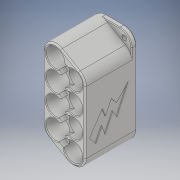
# Autodesk Inventor part: AUX_battery_pack
Saved by Autodesk Inventor 2019 (Build 230136000, 136)
## iProperties
Created: 2019-11-13
Part Number: AUX_battery_pack
Material: Generic
Document SubType Name: Modeling
Designer: steve
Density: 1 g/cm^3
Appearance: Default
Author: steve
Autodesk Inventor part; units mm, degrees
ref_plane "YZ Plane" through (0, 0, 0) normal (1, 0, 0) x (0, 1, 0)
ref_plane "XZ Plane" through (0, 0, 0) normal (0, 1, 0) x (-1, 0, 0)
ref_plane "XY Plane" through (0, 0, 0) normal (0, 0, 1) x (1, 0, 0)
sketch "Sketch1" plane through (0, 0, 0) normal (0, 0, 1) x (1, 0, 0)
  circle A0 centre (0, 60) radius 13.45
  circle A1 centre (0, 30) radius 13.45
  circle A2 centre (0, 0) radius 13.45
  circle A3 centre (0, -30) radius 13.45
  line L0 (0, 60) -> (0, -30) construction
  circle A4 centre (25.980762, 45) radius 13.45
  circle A5 centre (25.980762, 15) radius 13.45
  circle A6 centre (25.980762, -15) radius 13.45
  circle A7 centre (25.980762, -45) radius 13.45
  line L1 (25.980762, 45) -> (25.980762, -45) construction
  line L2 (-17.45, 60) -> (-17.45, -30)
  line L3 (43.430762, 45) -> (43.430762, -45)
  arc A8 (17.255762, -60.112143) -> (43.430762, -45) centre (25.980762, -45) ccw
  line L4 (8.725, 75.112143) -> (34.705762, 60.112143)
  line L5 (17.255762, -60.112143) -> (-8.725, -45.112143)
  arc A9 (43.430762, 45) -> (34.705762, 60.112143) centre (25.980762, 45) ccw
  arc A10 (8.725, 75.112143) -> (-17.45, 60) centre (0, 60) ccw
  arc A11 (-17.45, -30) -> (-8.725, -45.112143) centre (0, -30) ccw
  dimension "d0" = 30
  dimension "d1" = 30
  dimension "d2" = 30
  dimension "d3" = 30
  dimension "d4" = 30
  dimension "d5" = 30
  dimension "d6" = 26.9
  dimension "d7" = 30
  dimension "d8" = 30
  dimension "d10" = 17.45
  dimension "d11" = 17.45
  constraints: 13 end point, 12 centre point, 8 point on circle, 7 equal radius, 7 tangent, 4 point on line, 4 vertical, 1 coincident, 1 parallel
  measures "d0" distance of A1.centre L0.start
  measures "d1" distance of A2.centre A1.centre
  measures "d2" distance of L0.end A2.centre
  measures "d3" distance of A5.centre L1.start
  measures "d4" distance of A6.centre A5.centre
  measures "d5" distance of L1.end A6.centre
  measures "d6" diameter of A0
  measures "d7" distance of L1.start L0.start
  measures "d8" distance of A1.centre L1.start
  measures "d10" distance from line of L2 L0.start
  measures "d11" distance from line of L3 L1.start
extrude "Extrusion1" add sketch "Sketch1" along normal blind 70
sketch "Sketch2" plane through (0, 0, 0) normal (0, 0, -1) x (-1, 0, 0)
  line L0 (8.725, -45.112143) -> (-17.255762, -60.112143)
  arc A0 (8.725, -45.112143) -> (17.45, -30) centre (0, -30) ccw
  line L1 (17.45, 60) -> (17.45, -30)
  arc A1 (-43.430762, -45) -> (-17.255762, -60.112143) centre (-25.980762, -45) ccw
  line L2 (-43.430762, -45) -> (-43.430762, 45)
  arc A2 (-34.705762, 60.112143) -> (-43.430762, 45) centre (-25.980762, 45) ccw
  line L3 (-34.705762, 60.112143) -> (-8.725, 75.112143)
  arc A3 (17.45, 60) -> (-8.725, 75.112143) centre (0, 60) ccw
  point P0 (0, 0)
extrude "Extrusion2" add sketch "Sketch2" along normal blind 5
sketch "Sketch3" plane through (0, 0, -5) normal (0, 0, -1) x (-1, 0, 0)
  circle A0 centre (0, -30) radius 13.45
  circle A1 centre (-25.980762, -45) radius 13.45
  circle A2 centre (-25.980762, -15) radius 13.45
  circle A3 centre (0, 0) radius 13.45
  circle A4 centre (-25.980762, 15) radius 13.45
  circle A5 centre (-25.980762, 45) radius 13.45
  circle A6 centre (0, 30) radius 13.45
  circle A7 centre (0, 60) radius 13.45
  line L0 (0, -30) -> (-25.980762, -45) construction
  line L1 (-3.75, -23.504809) -> (-29.730762, -38.504809)
  line L2 (-22.230762, -51.495191) -> (3.75, -36.495191)
  arc A8 (3.75, -36.495191) -> (-3.75, -23.504809) centre (0, -30) ccw
  arc A9 (-29.730762, -38.504809) -> (-22.230762, -51.495191) centre (-25.980762, -45) ccw
  line L3 (-25.980762, -15) -> (0, 0) construction
  line L4 (-29.730762, -8.504809) -> (-3.75, 6.495191)
  line L5 (3.75, -6.495191) -> (-22.230762, -21.495191)
  arc A10 (-29.730762, -8.504809) -> (-22.230762, -21.495191) centre (-25.980762, -15) ccw
  arc A11 (3.75, -6.495191) -> (-3.75, 6.495191) centre (0, 0) ccw
  line L6 (-25.980762, 15) -> (0, 30) construction
  line L7 (-22.230762, 8.504809) -> (3.75, 23.504809)
  line L8 (-3.75, 36.495191) -> (-29.730762, 21.495191)
  arc A12 (-29.730762, 21.495191) -> (-22.230762, 8.504809) centre (-25.980762, 15) ccw
  arc A13 (3.75, 23.504809) -> (-3.75, 36.495191) centre (0, 30) ccw
  line L9 (-25.980762, 45) -> (0, 60) construction
  line L10 (-29.730762, 51.495191) -> (-3.75, 66.495191)
  line L11 (3.75, 53.504809) -> (-22.230762, 38.504809)
  arc A14 (-29.730762, 51.495191) -> (-22.230762, 38.504809) centre (-25.980762, 45) ccw
  arc A15 (3.75, 53.504809) -> (-3.75, 66.495191) centre (0, 60) ccw
  point P0 (-12.990381, -37.5)
  point P1 (-12.990381, -7.5)
  point P2 (-12.990381, 22.5)
  point P3 (-12.990381, 52.5)
  dimension "d16" = 15
  constraints: 32 end point, 16 point on circle, 16 tangent, 8 centre point, 7 parallel, 4 midpoint, 3 equal radius, 1 coincident
  measures "d16" distance between parallel lines of L1 L2
extrude "Extrusion3" cut sketch "Sketch3" against normal blind 8 contours L1 A8 L2 A0 | A0 L2 A1 L1 | A1 L2 A9 L1 | A2 L5 A10 L4 | A2 L4 A3 L5 | L4 A11 L5 A3 | A4 L7 A12 L8 | A4 L8 A6 L7 | L8 A13 L7 A6 | A5 L11 A14 L10 | A5 L10 A7 L11 | L10 A15 L11 A7 picked at (-4.12012, -31.767735) picked at (-21.936079, -43.065881) picked at (-21.936079, -13.065881) picked at (-4.12012, -1.767735) picked at (-21.936079, 16.934119) picked at (-4.12012, 28.232265) picked at (-21.936079, 46.934119) picked at (-4.12012, 58.232265)
sketch "Sketch5" plane through (0, 0, 70) normal (0, 0, 1) x (1, 0, 0)
  circle A0 centre (25.980762, 45) radius 13.45
  circle A1 centre (0, 30) radius 13.45
  circle A2 centre (25.980762, 15) radius 13.45
  circle A3 centre (25.980762, -15) radius 13.45
  circle A4 centre (0, -30) radius 13.45
  line L0 (25.980762, 45) -> (0, 30) construction
  line L1 (22.230762, 51.495191) -> (-3.75, 36.495191)
  line L2 (3.75, 23.504809) -> (29.730762, 38.504809)
  arc A5 (29.730762, 38.504809) -> (22.230762, 51.495191) centre (25.980762, 45) ccw
  arc A6 (-3.75, 36.495191) -> (3.75, 23.504809) centre (0, 30) ccw
  arc A7 (3.75, 66.495191) -> (-3.75, 53.504809) centre (0, 60) ccw
  line L3 (25.980762, 15) -> (0, 0) construction
  line L4 (22.230762, 21.495191) -> (-3.75, 6.495191)
  line L5 (3.75, -6.495191) -> (29.730762, 8.504809)
  arc A8 (29.730762, 8.504809) -> (22.230762, 21.495191) centre (25.980762, 15) ccw
  arc A9 (-3.75, 6.495191) -> (3.75, -6.495191) centre (0, 0) ccw
  line L6 (25.980762, -15) -> (0, -30) construction
  line L7 (22.230762, -8.504809) -> (-3.75, -23.504809)
  line L8 (3.75, -36.495191) -> (29.730762, -21.495191)
  arc A10 (29.730762, -21.495191) -> (22.230762, -8.504809) centre (25.980762, -15) ccw
  arc A11 (-3.75, -23.504809) -> (3.75, -36.495191) centre (0, -30) ccw
  point P0 (12.990381, 37.5)
  point P1 (12.990381, 7.5)
  point P2 (12.990381, -22.5)
  constraints: 24 end point, 12 point on circle, 12 tangent, 6 centre point, 4 parallel, 3 equal radius, 3 midpoint
extrude "Extrusion5" cut sketch "Sketch5" against normal blind 8 contours L1 A5 L2 A0 | A0 L2 A1 L1 | A1 L2 A6 L1 | L4 A8 L5 A2 | A2 L5 A9 L4 | L7 A10 L8 A3 | A3 L8 A4 L7 | A4 L8 A11 L7 picked at (21.860642, 43.232265) picked at (4.044683, 31.934119) picked at (21.860642, 13.232265) picked at (21.860642, -16.767735) picked at (4.044683, -28.065881)
sketch "Sketch6" plane through (0, 0, -5) normal (0, 0, -1) x (-1, 0, 0)
  arc A0 (17.45, 60) -> (-8.725, 75.112143) centre (0, 60) ccw
  line L0 (0, 77.45) -> (-25.980762, 77.45)
  line L1 (-43.430762, -45) -> (-43.430762, 45)
  line L2 (-43.430762, 60) -> (-43.430762, 45)
  arc A1 (-43.430762, -45) -> (-17.255762, -60.112143) centre (-25.980762, -45) ccw
  line L3 (-25.980762, -62.45) -> (0, -62.45)
  arc A2 (8.725, -45.112143) -> (17.45, -30) centre (0, -30) ccw
  line L4 (17.45, -45) -> (17.45, -30)
  arc A3 (0, -62.45) -> (17.45, -45) centre (0, -45) ccw
  arc A4 (-25.980762, 77.45) -> (-43.430762, 60) centre (-25.980762, 60) ccw
  arc A5 (17.45, 60) -> (-8.725, 75.112143) centre (0, 60) ccw
  circle A6 centre (-32.980762, 68) radius 3.5
  circle A7 centre (7, -53) radius 3.5
  arc A8 (-34.705762, 60.112143) -> (-43.430762, 45) centre (-25.980762, 45) ccw
  line L5 (-8.725, 75.112143) -> (-34.705762, 60.112143)
  line L6 (-17.255762, -60.112143) -> (8.725, -45.112143)
  point P0 (0, 0)
  dimension "d25" = 7
  dimension "d26" = 8
  dimension "d27" = 8
  dimension "d28" = 7
  dimension "d29" = 7
  constraints: 8 end point, 7 tangent, 6 point on circle, 4 centre point, 3 equal radius, 2 horizontal, 1 collinear, 1 perpendicular
  measures "d25" horizontal distance of A4.centre A6.centre
  measures "d26" vertical distance of A4.centre A6.centre
  measures "d27" vertical distance of A3.centre A7.centre
  measures "d28" horizontal distance of A3.centre A7.centre
  measures "d29" diameter of A6
extrude "Extrusion6" add sketch "Sketch6" against normal blind 8
chamfer "Chamfer1" distance 1 angle 45 6 edges at (12.9904, 77.45, 3) (38.3198, 72.339, 3) (43.4308, 52.5, 3) (-12.339, -57.339, 3) (12.9904, -62.45, 3) (-17.45, -37.5, 3)
chamfer "Chamfer2" distance 2 angle 45 16 edges at (-17.45, 15, 70) (-15.1121, -38.725, 70) (4.2654, -52.6121, 70) (34.7058, -60.1121, 70) (43.4308, 0, 70) (41.0929, 53.725, 70) (21.7154, 67.6121, 70) (-8.725, 75.1121, 70) (-17.45, 7.5, -5) (-12.339, 72.339, -5) (12.9904, 77.45, -5) (38.3198, 72.339, -5) (43.4308, 7.5, -5) (38.3198, -57.339, -5) (12.9904, -62.45, -5) (-12.339, -57.339, -5)
fillet "Fillet1" radius 1 11 edges at (12.5308, -45, 70) (-11.648, -36.725, 70) (-11.648, -6.725, 70) (33.0974, -26.413, 70) (26.4374, -1.5578, 70) (33.0974, 3.587, 70) (26.4374, 28.4422, 70) (-11.648, 23.275, 70) (-13.45, 60, 70) (33.0974, 33.587, 70) (26.4374, 58.4422, 70)
sketch "Sketch7" plane through (43.430762, 45, 2) normal (1, 0, 0) x (0, 0, -1)
  line L0 (-52.607783, -78.238394) -> (-61.826281, -67.020119)
  line L1 (-61.826281, -67.020119) -> (-43.228078, -39.325419)
  line L2 (-43.228078, -39.325419) -> (-38.644697, -50.847251)
  line L3 (-30.271785, -32.948873) -> (-22.700002, -42.051274)
  line L4 (-22.700002, -42.051274) -> (-5.868775, -23.837274)
  line L5 (-28.217884, -49.779066) -> (-22.387126, -60.267263)
  line L6 (-22.387126, -60.267263) -> (-5.868775, -23.837274)
  line L7 (-28.217884, -49.779066) -> (-39.286312, -73.570399)
  line L8 (-39.286312, -73.570399) -> (-43.874505, -60.51306)
  line L9 (-43.874505, -60.51306) -> (-52.607783, -78.238394)
  line L10 (-38.644697, -50.847251) -> (-30.271785, -32.948873)
  point P0 (2, -45)
  point P1 (23.5, -4.5)
  dimension "d39" = 33.36
  dimension "d40" = 14.52
  dimension "d41" = 19.76
  dimension "d42" = 13.84
  dimension "d43" = 26.24
  dimension "d44" = 19.76
  dimension "d45" = 12.4
  dimension "d46" = 11.84
  dimension "d47" = 24.8
  dimension "d48" = 40
  dimension "d49" = 12
  constraints: 22 end point
  measures "d39" distance of L0.end L1.end
  measures "d40" distance of L0.start L0.end
  measures "d41" distance of L8.end L0.start
  measures "d42" distance of L7.end L8.end
  measures "d43" distance of L5.start L7.end
  measures "d44" distance of L2.end L3.start
  measures "d45" distance of L1.end L2.end
  measures "d46" distance of L3.start L3.end
  measures "d47" distance of L3.end L4.end
  measures "d48" distance of L5.end L4.end
  measures "d49" distance of L5.start L5.end
extrude "Extrusion7" cut sketch "Sketch7" against normal blind 1
sketch "Sketch8" plane through (0, 0, 70) normal (0, 0, 1) x (1, 0, 0)
  arc A0 (5.91899, -17.922415) -> (13.41899, -30.912796) centre (0, -30) ccw
  arc A1 (20.061772, -27.077585) -> (12.561772, -14.087204) centre (25.980762, -15) ccw
  arc A2 (5.91899, 12.077585) -> (13.41899, -0.912796) centre (0, 0) ccw
  arc A3 (20.061772, 2.922415) -> (12.561772, 15.912796) centre (25.980762, 15) ccw
  arc A4 (5.91899, 42.077585) -> (13.41899, 29.087204) centre (0, 30) ccw
  arc A5 (20.061772, 32.922415) -> (12.561772, 45.912796) centre (25.980762, 45) ccw
  circle A6 centre (0, 60) radius 13.45
  circle A7 centre (25.980762, -45) radius 13.45
  arc A8 (22.230762, 38.504809) -> (29.730762, 51.495191) centre (25.980762, 45) ccw
  line L0 (0, 60) -> (25.980762, 45) construction
  line L1 (3.75, 66.495191) -> (29.730762, 51.495191)
  line L2 (22.230762, 38.504809) -> (-3.75, 53.504809)
  arc A9 (3.75, 66.495191) -> (-3.75, 53.504809) centre (0, 60) ccw
  arc A10 (22.230762, 38.504809) -> (29.730762, 51.495191) centre (25.980762, 45) ccw
  line L3 (0, 30) -> (25.980762, 15) construction
  line L4 (-3.75, 23.504809) -> (22.230762, 8.504809)
  line L5 (29.730762, 21.495191) -> (3.75, 36.495191)
  arc A11 (3.75, 36.495191) -> (-3.75, 23.504809) centre (0, 30) ccw
  arc A12 (22.230762, 8.504809) -> (29.730762, 21.495191) centre (25.980762, 15) ccw
  line L6 (0, 0) -> (25.980762, -15) construction
  line L7 (-3.75, -6.495191) -> (22.230762, -21.495191)
  line L8 (29.730762, -8.504809) -> (3.75, 6.495191)
  arc A13 (3.75, 6.495191) -> (-3.75, -6.495191) centre (0, 0) ccw
  arc A14 (22.230762, -21.495191) -> (29.730762, -8.504809) centre (25.980762, -15) ccw
  line L9 (0, -30) -> (25.980762, -45) construction
  line L10 (-3.75, -36.495191) -> (22.230762, -51.495191)
  line L11 (29.730762, -38.504809) -> (3.75, -23.504809)
  arc A15 (3.75, -23.504809) -> (-3.75, -36.495191) centre (0, -30) ccw
  arc A16 (22.230762, -51.495191) -> (29.730762, -38.504809) centre (25.980762, -45) ccw
  point P0 (12.990381, 52.5)
  point P1 (12.990381, 22.5)
  point P2 (12.990381, -7.5)
  point P3 (12.990381, -37.5)
  constraints: 32 end point, 16 point on circle, 16 tangent, 8 centre point, 5 parallel, 4 equal radius, 4 midpoint
extrude "Extrusion8" cut sketch "Sketch8" against normal blind 8 contours A6 L2 A9 L1 | A6 L1 A8 L2 | L11 A16 L10 A7 | A7 L10 A15 L11 | A11 L5 A12 L4 | A13 L8 A14 L7 picked at (4.044683, 58.065881) picked at (21.860642, -43.232265)
sketch "Sketch9" plane through (0, 0, -5) normal (0, 0, -1) x (-1, 0, 0)
  arc A0 (3.75, -36.495191) -> (-3.75, -23.504809) centre (0, -30) ccw
  arc A1 (-29.730762, -8.504809) -> (-22.230762, -21.495191) centre (-25.980762, -15) ccw
  arc A2 (3.75, 23.504809) -> (-3.75, 36.495191) centre (0, 30) ccw
  arc A3 (-29.730762, 51.495191) -> (-22.230762, 38.504809) centre (-25.980762, 45) ccw
  line L0 (0, -30) -> (-25.980762, -15) construction
  line L1 (3.75, -23.504809) -> (-22.230762, -8.504809)
  line L2 (-29.730762, -21.495191) -> (-3.75, -36.495191)
  arc A4 (-3.75, -36.495191) -> (3.75, -23.504809) centre (0, -30) ccw
  arc A5 (-22.230762, -8.504809) -> (-29.730762, -21.495191) centre (-25.980762, -15) ccw
  arc A6 (-29.730762, 21.495191) -> (-22.230762, 8.504809) centre (-25.980762, 15) ccw
  arc A7 (3.75, -6.495191) -> (-3.75, 6.495191) centre (0, 0) ccw
  line L3 (0, 0) -> (-25.980762, 15) construction
  line L4 (-3.75, -6.495191) -> (-29.730762, 8.504809)
  line L5 (-22.230762, 21.495191) -> (3.75, 6.495191)
  arc A8 (-3.75, -6.495191) -> (3.75, 6.495191) centre (0, 0) ccw
  arc A9 (-22.230762, 21.495191) -> (-29.730762, 8.504809) centre (-25.980762, 15) ccw
  line L6 (0, 30) -> (-25.980762, 45) construction
  line L7 (3.75, 36.495191) -> (-22.230762, 51.495191)
  line L8 (-29.730762, 38.504809) -> (-3.75, 23.504809)
  arc A10 (-3.75, 23.504809) -> (3.75, 36.495191) centre (0, 30) ccw
  arc A11 (-22.230762, 51.495191) -> (-29.730762, 38.504809) centre (-25.980762, 45) ccw
  point P0 (-12.990381, -22.5)
  point P1 (-12.990381, 7.5)
  point P2 (-12.990381, 37.5)
  constraints: 24 end point, 12 point on circle, 12 tangent, 6 centre point, 4 parallel, 3 equal radius, 3 midpoint
extrude "Extrusion9" cut sketch "Sketch9" against normal blind 8
equation "\"d1\" = d0"
equation "\"d2\" = d0"
equation "\"d3\" = d0"
equation "\"d4\" = d3"
equation "\"d5\" = d3"
equation "\"d11\" = d10"
equation "\"d27\" = d26"
equation "\"d28\" = d25"
equation "\"d39\" = 0.834 * d48"
equation "\"d40\" = 0.363 * d48"
equation "\"d41\" = 0.494 * d48"
equation "\"d42\" = 0.346 * d48"
equation "\"d43\" = 0.656 * d48"
equation "\"d44\" = 0.494 * d48"
equation "\"d45\" = 0.31 * d48"
equation "\"d46\" = 0.296 * d48"
equation "\"d47\" = 0.62 * d48"
equation "\"d49\" = 0.3 * d48"
body "Solid1"
